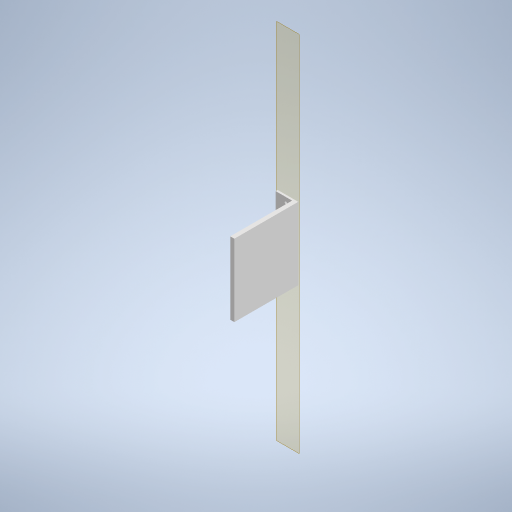
# Autodesk Inventor part: Front-Back Sensor Holds
Saved by Autodesk Inventor 2024 (Build 280153000, 153)
## iProperties
Created: 2024-01-19
Part Number: Front-Back Sensor Holds
Material: Generic
Document SubType Name: Modeling
Designer: Guru
Density: 1 g/cm^3
Appearance: Default
Author: Guru
Autodesk Inventor part; units mm, degrees
ref_plane "YZ Plane" through (0, 0, 0) normal (1, 0, 0) x (0, 1, 0)
ref_plane "XZ Plane" through (0, 0, 0) normal (0, 1, 0) x (-1, 0, 0)
ref_plane "XY Plane" through (0, 0, 0) normal (0, 0, 1) x (1, 0, 0)
ref_plane "Work Plane2" through (0, 0, 0) normal (0, 0, 1) x (1, 0, 0)
sketch "Sketch2" plane through (0, 0, 0) normal (0, 0, 1) x (1, 0, 0)
  line L0 (0, 0) -> (0, 406.4) projected
  line L1 (25.4, 0) -> (25.4, 406.4) projected
  circle A0 centre (12.7, 165.1) radius 1.5875 projected
  circle A1 centre (12.7, 190.5) radius 1.5875 projected
  circle A2 centre (12.7, 215.9) radius 1.5875 projected
  circle A3 centre (12.7, 241.3) radius 1.5875 projected
  line L2 (0, 158.75) -> (25.4, 158.75)
  line L3 (25.4, 158.75) -> (25.4, 247.65)
  line L4 (25.4, 247.65) -> (0, 247.65)
  line L5 (0, 247.65) -> (0, 158.75)
  point P0 (0, 158.75)
  point P1 (25.4, 247.65)
  point P2 (25.4, 158.75)
  point P3 (0, 247.65)
  dimension "d2" = 0
  dimension "d3" = 0
  dimension "d4" = 0
  dimension "d0" = 6.35
  dimension "d1" = 6.35
  constraints: 8 end point, 6 point on line, 5 horizontal, 4 vertical, 2 parallel, 1 perpendicular, 16 other
  measures "d0" distance from line of L2 A0.centre
  measures "d1" distance from line of L4 A3.centre
extrude "Extrusion1" add sketch "Sketch2" along normal blind 2.54
sketch "Sketch3" plane through (0, 0, 2.54) normal (0, 0, 1) x (1, 0, 0)
  line L0 (25.4, 158.75) -> (25.4, 247.65) projected
  line L1 (25.4, 247.65) -> (20.32, 247.65)
  line L2 (20.32, 247.65) -> (20.32, 158.75)
  line L3 (20.32, 158.75) -> (25.4, 158.75)
  line L4 (25.4, 158.75) -> (25.4, 247.65)
  point P0 (0, 0)
  dimension "d8" = 5.08
  dimension "d9" = 88.9
  constraints: 8 end point, 2 parallel, 1 horizontal, 1 perpendicular
  measures "d8" distance of L3.end L2.end
  measures "d9" distance of L2.end L1.end
extrude "Extrusion2" add sketch "Sketch3" along normal blind 76.2
body "Solid1"
